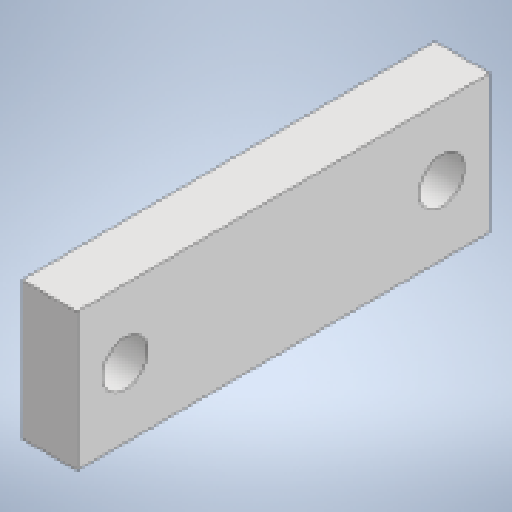
# Autodesk Inventor part: BF10_3030_Mount
Saved by Autodesk Inventor 2023 (Build 270158000, 158)
## iProperties
Created: 2022-04-29
Part Number: BF10_3030_Mount
Material: Generic
Document SubType Name: Modeling
Designer: plebbb
Density: 1 g/cm^3
Appearance: Default
Author: plebbb
Autodesk Inventor part; units mm, degrees
ref_plane "YZ Plane" through (0, 0, 0) normal (1, 0, 0) x (0, 1, 0)
ref_plane "XZ Plane" through (0, 0, 0) normal (0, 1, 0) x (-1, 0, 0)
ref_plane "XY Plane" through (0, 0, 0) normal (0, 0, 1) x (1, 0, 0)
sketch "Sketch1" plane through (0, 0, 0) normal (1, 0, 0) x (0, 1, 0)
  line L0 (0, 0) -> (20, 0)
  line L1 (20, 0) -> (20, -60)
  line L2 (20, -60) -> (0, -60)
  line L3 (0, -60) -> (0, 0)
  circle A0 centre (10, -7) radius 3.3
  circle A1 centre (10, -53) radius 3.3
  dimension "d0" = 20
  dimension "d1" = 60
  dimension "d2" = 6.6
  dimension "d3" = 6.6
  dimension "d4" = 46
  dimension "d5" = 10
  dimension "d6" = 7
  constraints: 8 end point, 2 centre point, 2 parallel, 1 horizontal, 1 perpendicular, 1 vertical alignment
  measures "d0" distance of L1.end L2.end
  measures "d1" distance of L0.end L1.end
  measures "d2" diameter of A0
  measures "d3" diameter of A1
  measures "d4" distance of A1.centre A0.centre
  measures "d5" horizontal distance of L0.end A0.centre
  measures "d6" vertical distance of L0.end A0.centre
extrude "Extrusion1" add sketch "Sketch1" along normal blind 8
body "Solid1"
